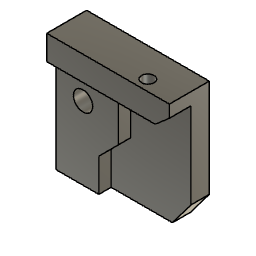
shape1 (Autodesk Fusion 360 design; units mm, degrees)
Autodesk Fusion 360 part; units mm, degrees
sketch "Sketch1" plane through (0, 0, 0) normal (0, 1, 0) x (1, 0, 0)
  line L0 (0, 0) -> (0, -200)
  line L1 (0, -200) -> (200, -200)
  line L2 (200, -200) -> (200, -40)
  line L3 (170, 0) -> (0, 0)
  line L4 (170, 0) -> (200, -40)
  line L5 (93.465, -147.4251) -> (198.1071, -147.4251)
  line L6 (93.465, -147.4251) -> (93.465, -145)
  constraint coincident L0.start L3.end
  constraint vertical L0
  constraint perpendicular L0 L1
  constraint perpendicular L1 L2
  constraint perpendicular L0 L3
  constraint perpendicular L0 L5
  constraint perpendicular L5 L6
extrude "Extrude1" add sketch "Sketch1" along normal blind 30 makes body 1
sketch "Sketch2" plane through (0, 0, 0) normal (0, 1, 0) x (1, 0, 0)
  line L0 (0, -160) -> (197.6402, -160)
  line L1 (197.6402, -160) -> (200, -160)
  line L2 (101.8607, -160) -> (101.8607, -85.8975)
  line L3 (70, -53.971) -> (70, 0)
  line L4 (101.8607, -85.8975) -> (70, -53.971)
  line L5 (0, -160) -> (0, 0)
  line L6 (0, 0) -> (70, 0)
  constraint horizontal L0
  constraint parallel L0 L1
  constraint coincident L0 L2.start
  constraint perpendicular L0 L2
  constraint perpendicular L0 L3
  constraint coincident L5.end L6.start
  constraint perpendicular L0 L5
  constraint perpendicular L3 L6
extrude "Extrude2" add sketch "Sketch2" against normal blind 20 separate body makes body 2
sketch "Sketch3" plane through (0, -20, 0) normal (0, -1, 0) x (1, 0, 0)
  line L0 (101.8607, 160) -> (0, 160)
  line L1 (0, 160) -> (0, 0)
  line L2 (0, 0) -> (70, 0)
  line L3 (70, 0) -> (70, 53.971)
  line L4 (70, 53.971) -> (101.8607, 85.8975)
  line L5 (101.8607, 85.8975) -> (101.8607, 160)
  line L6 (2.5338, 160) -> (176.8626, 160)
  line L7 (200, 160) -> (200, 200)
  line L8 (200, 200) -> (0, 200)
  line L9 (0, 200) -> (0, 160)
  line L10 (176.8626, 160) -> (200, 180)
  constraint coincident L0 L6.start
  constraint perpendicular L1 L6
  constraint perpendicular L6 L7
  constraint perpendicular L7 L8
  constraint coincident L0.end L1.start
  constraint perpendicular L0 L9
  constraint midpoint L7 L10.end
extrude "Extrude3" add sketch "Sketch3" against normal blind 20 contours L0 L6 L7 L8 L9 L10 bodies 1 2
sketch "Sketch4" plane through (0, -20, 0) normal (0, -1, 0) x (1, 0, 0)
  line L0 (0, 200) -> (0, 0)
  line L1 (0, 0) -> (70, 0)
  line L2 (70, 0) -> (70, 53.971)
  line L3 (70, 53.971) -> (101.8607, 85.8975)
  line L4 (101.8607, 85.8975) -> (101.8607, 160)
  line L5 (101.8607, 160) -> (176.8626, 160)
  line L6 (176.8626, 160) -> (200, 180)
  line L7 (200, 180) -> (200, 200)
  line L8 (200, 200) -> (0, 200)
  line L9 (-5.5994, 160) -> (173.5818, 160)
  line L10 (200, 180) -> (200, 200)
  line L11 (0, 200) -> (0, 160)
  constraint coincident L5 L9.end
  constraint perpendicular L0 L9
  constraint coincident L6.end L7.start
  constraint coincident L7.end L8.start
  constraint coincident L0.start L8.end
  constraint coincident L9 L11.end
  constraint coincident L0 L11.end
extrude "Extrude4" add sketch "Sketch4" along normal blind 15 contours L0 L5 L6 L7 L8 L9 L10 L11 bodies 1
sketch "Sketch5" plane through (0, -20, 0) normal (0, -1, 0) x (1, 0, 0)
  line L0 (101.8607, 160) -> (0, 160)
  line L1 (0, 160) -> (0, 0)
  line L2 (0, 0) -> (70, 0)
  line L3 (70, 0) -> (70, 53.971)
  line L4 (70, 53.971) -> (101.8607, 85.8975)
  line L5 (101.8607, 85.8975) -> (101.8607, 160)
  circle A0 centre (44.2368, 119.0792) radius 15.737
extrude "Extrude5" cut sketch "Sketch5" against normal blind 60 contours A0 bodies 1
sketch "Sketch6" plane through (0, 0, 160) normal (0, 0, -1) x (1, 0, 0)
  line L0 (101.8607, 20) -> (101.8607, 0)
  line L1 (101.8607, 0) -> (176.8626, 0)
  line L2 (176.8626, 0) -> (176.8626, 35)
  line L3 (176.8626, 35) -> (0, 35)
  line L4 (0, 35) -> (0, 20)
  line L5 (0, 20) -> (101.8607, 20)
  circle A0 centre (147.113, 17.2318) radius 10.2876
extrude "Extrude6" cut sketch "Sketch6" against normal blind 40 contours A0 bodies 1
